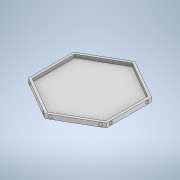
# Autodesk Inventor part: hexlight-bottom-led-module
Saved by Autodesk Inventor 2020 (Build 240168000, 168)
## iProperties
Created: 2019-10-02
Part Number: hexlight-bottom-led-module
Material: Generic
Document SubType Name: Modeling
Designer: Adam
Density: 1 g/cm^3
Appearance: Default
Author: Adam
Autodesk Inventor part; units mm, degrees
ref_plane "YZ Plane" through (0, 0, 0) normal (1, 0, 0) x (0, 1, 0)
ref_plane "XZ Plane" through (0, 0, 0) normal (0, 1, 0) x (-1, 0, 0)
ref_plane "XY Plane" through (0, 0, 0) normal (0, 0, 1) x (1, 0, 0)
sketch "Sketch1" plane through (0, 0, 0) normal (0, 1, 0) x (-1, 0, 0)
  line L0 (73.6122, 42.5) -> (73.6122, -42.5)
  line L1 (73.6122, -42.5) -> (0, -85)
  line L2 (0, -85) -> (-73.6122, -42.5)
  line L3 (-73.6122, -42.5) -> (-73.6122, 42.5)
  line L4 (-73.6122, 42.5) -> (0, 85)
  line L5 (0, 85) -> (73.6122, 42.5)
  point P0 (0, 0)
  point P1 (0, 0)
  dimension "d1" = 0
  dimension "d2" = 85
  constraints: 12 end point, 1 coincident, 13 other
  measures "d1" horizontal distance of point (0, 0) L4.end
  measures "d2" distance of L0.start L0.end
extrude "Extrusion1" add sketch "Sketch1" along normal blind 8
sketch "Sketch2" plane through (0, 8, 0) normal (0, 1, 0) x (1, 0, 0)
  line L0 (-69.282, -40) -> (-69.282, 40)
  line L1 (-69.282, 40) -> (0, 80)
  line L2 (0, 80) -> (69.282, 40)
  line L3 (69.282, 40) -> (69.282, -40)
  line L4 (69.282, -40) -> (0, -80)
  line L5 (0, -80) -> (-69.282, -40)
  point P0 (0, 0)
  point P1 (0, 0)
  dimension "d5" = 0
  dimension "d6" = 80
  constraints: 12 end point, 1 coincident, 13 other
  measures "d5" horizontal distance of point (0, 0) L4.end
  measures "d6" distance of L0.start L0.end
extrude "Extrusion2" cut sketch "Sketch2" against normal blind 6
sketch "Sketch3" plane through (73.6122, 0, 42.5) normal (0.5, 0, 0.8660254) x (0.8660254, 0, -0.5)
  line L0 (-85, 0) -> (0, 0) projected
  line L1 (-85, 0) -> (-85, 8) projected
  line L2 (0, 0) -> (0, 8) projected
  point P0 (-42.5, 0)
  point P1 (-77, 4)
  point P2 (-8, 4)
  dimension "d9" = 4
  dimension "d10" = 8
  dimension "d11" = 0
  dimension "d12" = 8
  measures "d9" distance from line of L0 point (-77, 4)
  measures "d10" distance from line of L1 point (-77, 4)
  measures "d11" vertical distance of point (-77, 4) point (-8, 4)
  measures "d12" distance from line of L2 point (-8, 4)
hole "Hole1" at (6.9282, 4, 81) at (66.684, 4, 46.5) direction (-0.5, 0, -0.8660254) diameter 6 depth 1.5 tip angle 118
pattern_circular "Circular Pattern1" count 6 over 360 about axis through (0, -10, 0) along (0, 1, 0) of "Hole1"
body "Solid1"
